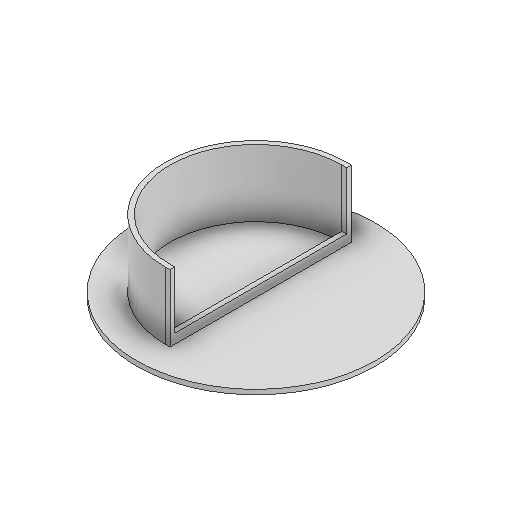
# Autodesk Inventor part: Shield_WeldSupport
Saved by Autodesk Inventor 2026.2 (Build 302298000, 298)
## iProperties
Created: 2026-06-09
Part Number: Shield_WeldSupport
Material: Generic
Document SubType Name: Modeling
Designer: zetsu
Density: 1 g/cm^3
Appearance: Default
Author: zetsu
Autodesk Inventor part; units mm, degrees
ref_plane "YZ Plane" through (0, 0, 0) normal (1, 0, 0) x (0, 1, 0)
ref_plane "XZ Plane" through (0, 0, 0) normal (0, 1, 0) x (-1, 0, 0)
ref_plane "XY Plane" through (0, 0, 0) normal (0, 0, 1) x (1, 0, 0)
sketch "スケッチ1" plane through (0, 0, 0) normal (0, 1, 0) x (-1, 0, 0)
  arc A0 (0, -19) -> (0, 19) centre (0, 0) ccw
  line L0 (0, 19) -> (-1, 19)
  line L1 (-1, 19) -> (-1, -19)
  line L2 (-1, -19) -> (0, -19)
  dimension "d0" = 19
  dimension "d1" = 1
  dimension "d2" = 38
  constraints: 6 end point, 3 point on circle, 2 perpendicular, 1 centre point, 1 coincident, 1 horizontal
  measures "d0" radius of A0
  measures "d1" distance of L0.start L0.end
  measures "d2" distance of L0.end L1.end
extrude "押し出し1" add sketch "スケッチ1" along normal blind 15
sketch "スケッチ2" plane through (0, 15, 0) normal (0, 1, 0) x (1, 0, 0)
  arc A0 (0, 18) -> (0, -18) centre (0, 0) ccw
  line L0 (0, -18) -> (0, 18)
  dimension "d5" = 18
  constraints: 2 end point, 2 point on circle, 1 centre point, 1 coincident, 1 vertical
  measures "d5" radius of A0
extrude "押し出し2" cut sketch "スケッチ2" against normal blind 14
sketch "スケッチ3" plane through (0, 15, 0) normal (0, 1, 0) x (1, 0, 0)
  line L0 (0, 18) -> (0, -18) projected
  line L1 (0, -18) -> (2.1384, -18)
  line L2 (2.1384, -18) -> (2.1384, 18)
  line L3 (2.1384, 18) -> (0, 18)
  line L4 (0, 18) -> (0, -18)
  point P0 (0, 0)
  dimension "d13" = 36
  constraints: 8 end point, 2 parallel, 1 horizontal, 1 perpendicular
  measures "d13" distance of L1.end L2.end
extrude "押し出し3" cut sketch "スケッチ3" against normal blind 12
sketch "スケッチ4" plane through (0, 0, 0) normal (0, -1, 0) x (1, 0, 0)
  circle A0 centre (0, 0) radius 25
  dimension "d10" = 50
  constraints: 1 centre point, 1 coincident
  measures "d10" diameter of A0
extrude "押し出し4" add sketch "スケッチ4" against normal blind 1
